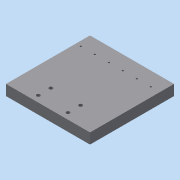
# Autodesk Inventor part: base of car 2
Saved by Autodesk Inventor 2015 (Build 190159000, 159)
## iProperties
Created: 2015-06-24
Part Number: base of car 2
Material: Generic
Document SubType Name: Modeling
Designer: Rahul
Density: 1 g/cm^3
Appearance: Default
Author: Rahul
Autodesk Inventor part; units mm, degrees
ref_plane "YZ Plane" through (0, 0, 0) normal (1, 0, 0) x (0, 1, 0)
ref_plane "XZ Plane" through (0, 0, 0) normal (0, 1, 0) x (-1, 0, 0)
ref_plane "XY Plane" through (0, 0, 0) normal (0, 0, 1) x (1, 0, 0)
sketch "Sketch1" plane through (0, 0, 0) normal (0, 1, 0) x (-1, 0, 0)
  line L0 (97.79, -118.745) -> (-54.61, -118.745)
  line L1 (-54.61, -118.745) -> (-54.61, 33.655)
  line L2 (-54.61, 33.655) -> (97.79, 33.655)
  line L3 (97.79, 33.655) -> (97.79, -118.745)
  point P0 (0, 0)
  dimension "d0" = 152.4
  dimension "d1" = 152.4
  constraints: 8 end point, 2 parallel, 1 horizontal, 1 perpendicular
  measures "d0" distance of L0.start L0.end
  measures "d1" distance of L0.end L1.end
extrude "Extrusion1" add sketch "Sketch1" against normal blind 19.05
sketch "Sketch2" plane through (0, 0, 0) normal (0, 1, 0) x (1, 0, 0)
  circle A0 centre (-88.8746, 93.345) radius 1.5875
  line L0 (-97.79, 118.745) -> (54.61, 118.745) projected
  line L1 (-97.79, -33.655) -> (-97.79, 118.745) projected
  point P0 (0, 0)
  dimension "d4" = 25.4
  dimension "d5" = 3.175
  dimension "d6" = 8.9154
  constraints: 1 centre point
  measures "d4" distance from line of A0.centre L0
  measures "d5" diameter of A0
  measures "d6" distance from line of L1 A0.centre
extrude "Extrusion2" cut sketch "Sketch2" against normal blind 19.05
pattern_linear "Rectangular Pattern1" count 6 spacing 25.4 along (1, 0, 0) of "Extrusion2"
sketch "Sketch3" plane through (0, 0, 0) normal (0, 1, 0) x (1, 0, 0)
  circle A0 centre (3.4544, -22.352) radius 3.2258
  line L0 (54.61, -33.655) -> (-97.79, -33.655) projected
  line L1 (54.61, 118.745) -> (54.61, -33.655) projected
  circle A1 centre (-50.4698, -22.352) radius 3.2258
  circle A2 centre (3.4544, 0.5588) radius 3.2258
  circle A3 centre (-50.4698, 0.5588) radius 3.2258
  point P0 (0, 0)
  dimension "d12" = 11.303
  dimension "d13" = 51.1556
  dimension "d14" = 6.4516
  dimension "d15" = 53.9242
  dimension "d16" = 22.9108
  dimension "d17" = 6.4516
  constraints: 4 centre point
  measures "d12" distance from line of L0 A0.centre
  measures "d13" distance from line of L1 A0.centre
  measures "d14" diameter of A0
  measures "d15" distance of A1.centre A0.centre
  measures "d16" distance of A2.centre A0.centre
  measures "d17" diameter of A2
extrude "Extrusion3" cut sketch "Sketch3" against normal blind 25.4
equation "\"d17\" = d14"
body "Solid1"
